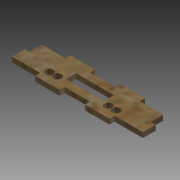
# Autodesk Inventor part: ShortMiddleStructure
Saved by Autodesk Inventor 2012 (Build 160160000, 160)
## iProperties
Created: 2014-07-01
Part Number: ShortMiddleStructure
Material: Default
Document SubType Name: Modeling
Designer: Laurent
Density: 1 g/cm^3
Author: Laurent
Autodesk Inventor part; units mm, degrees
ref_plane "YZ Plane" through (0, 0, 0) normal (1, 0, 0) x (0, 1, 0)
ref_plane "XZ Plane" through (0, 0, 0) normal (0, 1, 0) x (-1, 0, 0)
ref_plane "XY Plane" through (0, 0, 0) normal (0, 0, 1) x (1, 0, 0)
sketch "Sketch1" plane through (0, 0, 0) normal (0, 0, 1) x (1, 0, 0)
  line L0 (-52, 14) -> (52, 14)
  line L1 (52, 14) -> (52, -14)
  line L2 (52, -14) -> (-52, -14)
  line L3 (-52, -14) -> (-52, 14)
  point P0 (0, 0)
  dimension "d0" = 104
  dimension "d1" = 28
  dimension "d2" = 52
  dimension "d3" = 14
  constraints: 8 end point, 2 parallel, 1 horizontal, 1 perpendicular
  measures "d0" distance of L1.end L2.end
  measures "d1" distance between parallel lines of L0 L2
  measures "d2" distance from line of L3 point (0, 0)
  measures "d3" distance from line of L0 point (0, 0)
extrude "Base" add sketch "Sketch1" along normal blind 4
sketch "Sketch2" plane through (0, 0, 4) normal (0, 0, 1) x (1, 0, 0)
  line L0 (52, 14) -> (52, -14) projected
  line L1 (-52, 14) -> (52, 14) projected
  line L2 (-52, -14) -> (-52, 14) projected
  line L3 (52, -14) -> (-52, -14) projected
  line L4 (-52, 14) -> (-29.5, 14)
  line L5 (-29.5, 14) -> (-29.5, 10)
  line L6 (-29.5, 10) -> (-52, 10)
  line L7 (-52, 10) -> (-52, 14)
  line L8 (-52, -10) -> (-29.5, -10)
  line L9 (-29.5, -10) -> (-29.5, -14)
  line L10 (-29.5, -14) -> (-52, -14)
  line L11 (-52, -14) -> (-52, -10)
  line L12 (29.5, -10) -> (52, -10)
  line L13 (52, -10) -> (52, -14)
  line L14 (52, -14) -> (29.5, -14)
  line L15 (29.5, -14) -> (29.5, -10)
  line L16 (29.5, 14) -> (52, 14)
  line L17 (52, 14) -> (52, 10)
  line L18 (52, 10) -> (29.5, 10)
  line L19 (29.5, 10) -> (29.5, 14)
  line L20 (-10, 14) -> (10, 14)
  line L21 (10, 14) -> (10, 10)
  line L22 (10, 10) -> (-10, 10)
  line L23 (-10, 10) -> (-10, 14)
  line L24 (-10, -10) -> (10, -10)
  line L25 (10, -10) -> (10, -14)
  line L26 (10, -14) -> (-10, -14)
  line L27 (-10, -14) -> (-10, -10)
  point P0 (0, 0)
  dimension "d26" = 22.5
  dimension "d27" = 4
  dimension "d28" = 22.5
  dimension "d29" = 4
  dimension "d30" = 22.5
  dimension "d31" = 4
  dimension "d32" = 22.5
  dimension "d33" = 4
  dimension "d34" = 20
  dimension "d35" = 4
  dimension "d36" = 20
  dimension "d37" = 4
  dimension "d38" = 0
  dimension "d39" = 0
  dimension "d40" = 0
  dimension "d41" = 10
  dimension "d42" = 0
  dimension "d43" = 0
  dimension "d44" = 0
  dimension "d45" = 0
  dimension "d46" = 10
  dimension "d47" = 0
  dimension "d48" = 0
  dimension "d49" = 4
  constraints: 48 end point, 12 parallel, 6 horizontal, 6 perpendicular
  measures "d26" distance of L5.end L6.end
  measures "d27" distance of L4.end L5.end
  measures "d28" distance of L9.end L10.end
  measures "d29" distance of L8.end L9.end
  measures "d30" distance of L13.end L14.end
  measures "d31" distance of L12.end L13.end
  measures "d32" distance of L17.end L18.end
  measures "d33" distance of L16.end L17.end
  measures "d34" distance of L21.end L22.end
  measures "d35" distance of L20.end L21.end
  measures "d36" distance of L25.end L26.end
  measures "d37" distance of L24.end L25.end
  measures "d38" distance between parallel lines of L1 L4
  measures "d39" distance between parallel lines of L2 L7
  measures "d40" distance between parallel lines of L1 L20
  measures "d41" distance from line of point (0, 0) L23
  measures "d42" distance between parallel lines of L1 L16
  measures "d43" distance between parallel lines of L0 L17
  measures "d44" distance between parallel lines of L3 L10
  measures "d45" distance between parallel lines of L2 L11
  measures "d46" distance from line of point (0, 0) L27
  measures "d47" distance between parallel lines of L0 L13
  measures "d48" distance between parallel lines of L3 L14
  measures "d49" distance between parallel lines of L3 L24
extrude "PlatformsPattern" cut sketch "Sketch2" against normal blind 4 contours L0 L18 L19 L1 | L0 L3 L15 L12 | L21 L22 L23 L1 | L5 L6 L2 L1 | L3 L27 L24 L25 | L3 L2 L8 L9
sketch "Sketch3" plane through (0, 0, 4) normal (0, 0, 1) x (1, 0, 0)
  line L0 (52, 10) -> (52, -10) projected
  line L1 (52, 10) -> (29.5, 10) projected
  line L2 (-29.5, 10) -> (-52, 10) projected
  line L3 (-52, -10) -> (-52, 10) projected
  line L4 (-52, 10) -> (-48, 10)
  line L5 (-48, 10) -> (-48, 0)
  line L6 (-48, 0) -> (-52, 0)
  line L7 (-52, 0) -> (-52, 10)
  line L8 (48, 10) -> (52, 10)
  line L9 (52, 10) -> (52, 0)
  line L10 (52, 0) -> (48, 0)
  line L11 (48, 0) -> (48, 10)
  point P0 (0, 0)
  dimension "d52" = 4
  dimension "d53" = 10
  dimension "d54" = 4
  dimension "d55" = 10
  dimension "d56" = 0
  dimension "d57" = 0
  dimension "d58" = 0
  dimension "d59" = 0
  constraints: 16 end point, 4 parallel, 2 horizontal, 2 perpendicular
  measures "d52" distance of L5.end L6.end
  measures "d53" distance of L4.end L5.end
  measures "d54" distance of L10.start L10.end
  measures "d55" distance of L9.start L10.start
  measures "d56" distance between parallel lines of L3 L7
  measures "d57" distance between parallel lines of L2 L4
  measures "d58" distance between parallel lines of L0 L9
  measures "d59" distance between parallel lines of L1 L8
extrude "Sleeves" cut sketch "Sketch3" against normal blind 4
sketch "Sketch4" plane through (0, 0, 4) normal (0, 0, 1) x (1, 0, 0)
  line L0 (-15, 4) -> (15, 4)
  line L1 (15, 4) -> (15, -4)
  line L2 (15, -4) -> (-15, -4)
  line L3 (-15, -4) -> (-15, 4)
  point P0 (0, 0)
  dimension "d62" = 30
  dimension "d63" = 8
  dimension "d66" = 4
  dimension "d72" = 15
  constraints: 8 end point, 2 parallel, 1 horizontal, 1 perpendicular
  measures "d62" distance of L1.end L2.end
  measures "d63" distance of L0.end L1.end
  measures "d66" distance from line of point (0, 0) L0
  measures "d72" distance from line of point (0, 0) L3
extrude "Cabling" cut sketch "Sketch4" against normal blind 4
sketch "Sketch5" plane through (0, 0, 4) normal (0, 0, 1) x (1, 0, 0)
  line L0 (15, 4) -> (15, -4) projected
  line L1 (52, 0) -> (48, 0) projected
  line L2 (29.5, -10) -> (52, -10) projected
  line L3 (52, 0) -> (52, -10) projected
  line L4 (0, 13.359) -> (0, -17.1065) construction
  point P0 (0, 0)
  point P1 (20.08, -5.5)
  point P2 (26.43, -5.5)
  point P3 (-20.08, -5.5)
  point P4 (-26.43, -5.5)
  dimension "d75" = 5.08
  dimension "d76" = 6.35
  dimension "d78" = 4.5
  dimension "d79" = 5.5
  constraints: 2 end point, 2 symmetric about line, 1 parallel
  measures "d75" distance from line of L0 point (20.08, -5.5)
  measures "d76" distance of point (26.43, -5.5) point (20.08, -5.5)
  measures "d78" distance from line of L2 point (20.08, -5.5)
  measures "d79" distance from line of point (26.43, -5.5) L1
hole "ESCCutout" at (20.08, -5.5, 4) at (26.43, -5.5, 4) at (-20.08, -5.5, 4) at (-26.43, -5.5, 4) direction (0, 0, -1) diameter 6 end through all
body "Solid1"
